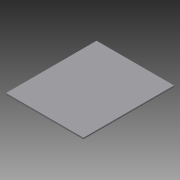
# Autodesk Inventor part: Flat Board
Saved by Autodesk Inventor 2014 (Build 180170000, 170)
## iProperties
Created: 2014-01-21
Part Number: Flat Board
Material: Generic
Document SubType Name: Modeling
Designer: NilesStanton
Density: 1 g/cm^3
Appearance: Default
Author: NilesStanton
Autodesk Inventor part; units mm, degrees
ref_plane "YZ Plane" through (0, 0, 0) normal (1, 0, 0) x (0, 1, 0)
ref_plane "XZ Plane" through (0, 0, 0) normal (0, 1, 0) x (-1, 0, 0)
ref_plane "XY Plane" through (0, 0, 0) normal (0, 0, 1) x (1, 0, 0)
sketch "Sketch1" plane through (0, 0, 0) normal (0, 1, 0) x (-1, 0, 0)
  line L0 (0, 0) -> (0, 438.15)
  line L1 (0, 438.15) -> (374.65, 438.15)
  line L2 (374.65, 438.15) -> (374.65, 0)
  line L3 (374.65, 0) -> (0, 0)
  dimension "d0" = 438.15
  dimension "d1" = 374.65
  constraints: 8 end point, 2 parallel, 1 perpendicular, 1 vertical
  measures "d0" distance of L1.end L2.end
  measures "d1" distance of L2.end L0.start
extrude "Extrusion1" add sketch "Sketch1" along normal blind 6.35
body "Solid1"
